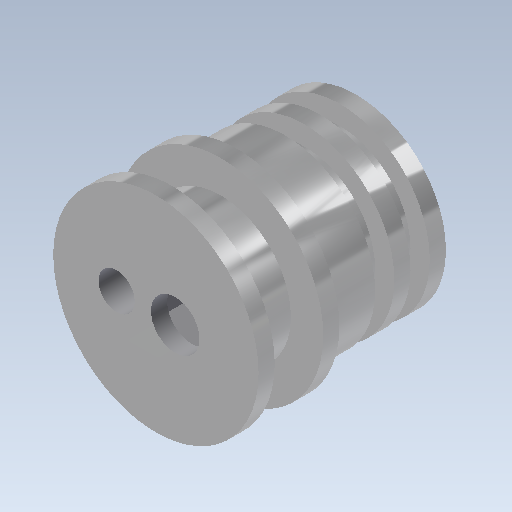
# Autodesk Inventor part: battery_cap
Saved by Autodesk Inventor 2020 (Build 240168000, 168)
## iProperties
Created: 2016-11-18
Part Number: battery_cap
Material: Generic
Document SubType Name: Modeling
Designer: jous
Density: 1 g/cm^3
Appearance: Default
Mass: 61.2111 g
Surface Area: 177.209 cm^2
Volume: 61.2111 cm^3
tube_ID: 44.450 mm
tube_OD: 50.800 mm
sheet: 4.000 mm
Author: jous
Autodesk Inventor part; units mm, degrees
ref_plane "YZ Plane" through (0, 0, 0) normal (1, 0, 0) x (0, 1, 0)
ref_plane "XZ Plane" through (0, 0, 0) normal (0, 1, 0) x (-1, 0, 0)
ref_plane "XY Plane" through (0, 0, 0) normal (0, 0, 1) x (1, 0, 0)
sketch "Sketch2" plane through (0, 0, 0) normal (0, 0, 1) x (1, 0, 0)
  circle A0 centre (0, 0) radius 22.225
  dimension "d4" = 44.45
  constraints: 1 centre point, 1 coincident
  measures "d4" diameter of A0
extrude "Extrusion2" add sketch "Sketch2" along normal blind 4
sketch "Sketch3" plane through (0, 0, 4) normal (0, 0, 1) x (1, 0, 0)
  circle A0 centre (0, 0) radius 22.225 projected
  circle A1 centre (0, 0) radius 17.4625
  dimension "d7" = 34.925
  constraints: 1 centre point, 1 coincident
  measures "d7" diameter of A1
extrude "Extrusion3" add sketch "Sketch3" along normal blind 4.7625 contours A1
sketch "Sketch4" plane through (0, 0, 8.7625) normal (0, 0, 1) x (1, 0, 0)
  circle A0 centre (0, 0) radius 17.4625 projected
  circle A1 centre (0, 0) radius 22.225
  dimension "d10" = 44.45
  constraints: 1 centre point, 1 coincident
  measures "d10" diameter of A1
extrude "Extrusion4" add sketch "Sketch4" along normal blind 4 contours A0 | A1
sketch "Sketch5" plane through (0, 0, 12.7625) normal (0, 0, 1) x (1, 0, 0)
  circle A0 centre (0, 0) radius 22.225 projected
  circle A1 centre (0, 0) radius 17.4625
  dimension "d13" = 34.925
  constraints: 1 centre point, 1 coincident
  measures "d13" diameter of A1
extrude "Extrusion5" add sketch "Sketch5" along normal blind 4.7625 contours A1
sketch "Sketch6" plane through (0, 0, 17.525) normal (0, 0, 1) x (1, 0, 0)
  circle A0 centre (0, 0) radius 17.4625 projected
  circle A1 centre (0, 0) radius 22.225
  dimension "d16" = 44.45
  constraints: 1 centre point, 1 coincident
  measures "d16" diameter of A1
extrude "Extrusion6" add sketch "Sketch6" along normal blind 12 contours A0 | A1
sketch "Sketch7" plane through (0, 0, 29.525) normal (0, 0, 1) x (1, 0, 0)
  circle A0 centre (0, 0) radius 22.225 projected
  circle A1 centre (0, 0) radius 25.4
  dimension "d19" = 50.8
  constraints: 1 centre point, 1 coincident
  measures "d19" diameter of A1
extrude "Extrusion7" add sketch "Sketch7" along normal blind 4 contours A0 | A1
sketch "Sketch8" plane through (0, 0, 33.525) normal (0, 0, 1) x (1, 0, 0)
  circle A0 centre (0, 0) radius 25.4 projected
  circle A1 centre (0, 0) radius 17.4
  dimension "d22" = 34.8
  constraints: 1 centre point, 1 coincident
  measures "d22" diameter of A1
extrude "Extrusion8" add sketch "Sketch8" along normal blind 12 contours A1
sketch "Sketch Main" plane through (0, 0, 45.525) normal (0, 0, 1) x (1, 0, 0)
  circle A0 centre (0, 0) radius 17.4 projected
  circle A1 centre (0, 0) radius 25.4
  line L0 (-17.4, 0) -> (17.4, 0) construction
  circle A2 centre (-9.7141, 0) radius 2.75
  circle A3 centre (-9.7141, 0) radius 4.5
  circle A4 centre (4.7812, 0) radius 6
  circle A5 centre (4.7812, 0) radius 9 construction
  circle A6 centre (4.7812, 0) radius 10 construction
  line L1 (13.4415, 5) -> (13.4415, -5)
  line L2 (13.4415, -5) -> (4.7812, -10)
  line L3 (4.7812, -10) -> (-3.879, -5)
  line L4 (-3.879, -5) -> (-3.879, 5)
  line L5 (-3.879, 5) -> (4.7812, 10)
  line L6 (4.7812, 10) -> (13.4415, 5)
  circle A7 centre (4.7812, 0) radius 1.5
  dimension "d51" = 20
  dimension "d25" = 50.8
  dimension "d39" = 5.5
  dimension "d40" = 9
  dimension "d41" = 12
  dimension "d42" = 18
  dimension "d56" = 3
  constraints: 14 end point, 6 centre point, 6 coincident, 2 point on circle, 2 point on line, 1 horizontal, 1 midpoint, 1 perpendicular, 16 other
  measures "d25" diameter of A1
  measures "d39" diameter of A2
  measures "d40" diameter of A3
  measures "d41" diameter of A4
  measures "d42" diameter of A5
  measures "d56" diameter of A7
extrude "Extrusion9" add sketch "Sketch Main" along normal blind 4 contours A0 | A1 | A2 | A3 | A4 | L1 L2 L3 L4 L5 L6 | A7
extrude "Extrusion13" cut sketch "Sketch Main" along normal blind 4 and the other way blind 16 contours A2 | A3
extrude "Extrusion14" cut sketch "Sketch Main" against normal through all contours A2
extrude "Extrusion15" cut sketch "Sketch Main" against normal blind 12 contours A4 | L1 L2 L3 L4 L5 L6 | A7
extrude "Extrusion16" cut sketch "Sketch Main" along normal through all contours A4 | A7
extrude "Extrusion17" cut sketch "Sketch Main" against normal through all contours A7
sketch "Sketch11" plane through (0, 0, 0) normal (0, 0, -1) x (-1, 0, 0)
  circle A0 centre (9.7141, 0) radius 2.75 projected
  circle A1 centre (9.7141, 0) radius 4.5
  dimension "d59" = 9
  constraints: 1 centre point, 1 coincident
  measures "d59" diameter of A1
extrude "Extrusion18" cut sketch "Sketch11" against normal blind 20 contours A0 | A1
body "Solid2"
